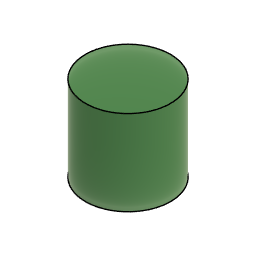
TrueTip Assembly (Autodesk Fusion 360 archive; units mm, degrees)
design "Traceline Dummy"
Autodesk Fusion 360 part; units mm, degrees
(part 1 of 3)
sketch "Sketch1" plane through (0, 0, 0) normal (0, 0, 1) x (1, 0, 0)
  circle A0 centre (0, 0) radius 0.05
  dimension "d1" = 0.1
  constraint coincident A0.centre origin
  measures "d1" diameter of A0
extrude "Extrude1" add sketch "Sketch1" along normal blind 0.1

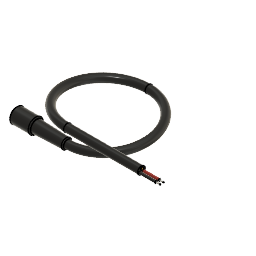
design "PE2 - 3-Pin Male Waterproof Connector (cut, coiled)"
Autodesk Fusion 360 part; units mm, degrees
sketch "Sketch1" plane through (0, 0, 0) normal (1, 0, 0) x (0, 1, 0)
  circle A0 centre (0, 0) radius 3.683
  circle A1 centre (0, 0) radius 3.175
  dimension "d1" = 7.366
  dimension "d2" = 6.35
  constraint coincident A0.centre A1.centre
  constraint concentric A0 A1
  measures "d1" diameter of A0
  measures "d2" diameter of A1
extrude "Extrude1" add sketch "Sketch1" along normal blind 10 contours A0 | A1 makes body 1
extrude "Extrude2" cut sketch "Sketch1" along normal blind 8 contours A1 bodies 1
sketch "Sketch2" plane through (0, 0, 0) normal (0, 1, 0) x (1, 0, 0)
  line L0 (10, 0) -> (10, -3)
  line L1 (10, -3) -> (25, -2.5)
  line L2 (25, -2.5) -> (25, 0)
  line L3 (25, 0) -> (10, 0)
  dimension "d7" = 3
  dimension "d46" = 15
  dimension "d47" = 88.091
  dimension "d48" = 10
  constraint vertical L0
  constraint vertical L2
  constraint perpendicular L0 L3
  constraint horizontal origin L0.start
  measures "d7" distance of L0.start L0.end
  measures "d46" distance of L0 L2
  measures "d47" angle of L0 L1
  measures "d48" distance of origin L0
revolve "Revolve1" add sketch "Sketch2" angle 360 about axis through (1.75, 0, 0) along (1, 0, 0) bodies 1
fillet "Fillet1" radius 0.5 3 edges at (0, -3.4338, -1.3318) (10, -3.4338, -1.3318) (25, -0.904, -2.3308) on bodies 1
sketch "Sketch4" plane through (8, 0, 0) normal (1, 0, 0) x (0, 1, 0)
  line L0 (0, 1.5) -> (-1.299, -0.75) construction
  line L1 (-1.299, -0.75) -> (1.299, -0.75) construction
  line L2 (1.299, -0.75) -> (0, 1.5) construction
  circle A0 centre (0, 1.5) radius 0.5
  circle A1 centre (-1.299, -0.75) radius 0.5
  circle A2 centre (1.299, -0.75) radius 0.5
  dimension "d15" = 1.5
  dimension "d16" = 1
  dimension "d17" = 1
  dimension "d18" = 1
  constraint coincident L0.start L2.end
  constraint coincident L0.end L1.start
  constraint coincident L1.end L2.start
  constraint horizontal L1
  measures "d15" distance of L0.start origin
  measures "d16" diameter of A0
  measures "d17" diameter of A1
  measures "d18" diameter of A2
extrude "Extrude4" add sketch "Sketch4" against normal blind 8 separate body makes body 2 at (2.6667, 0.4975, 1.4502) makes body 3 at (2.6667, 1.7966, -0.7998) makes body 4 at (2.6667, -0.8015, -0.7998)
fillet "Fillet2" radius 0.1 3 edges at (0, -0.4662, 1.6808) (0, 0.8329, -0.5692) (0, -1.7652, -0.5692) on bodies 2 3 4
sketch "Sketch3" plane through (25, 0, 0) normal (1, 0, 0) x (0, 1, 0)
  circle A0 centre (0, 0) radius 1.905
  circle A1 centre (0, 0) radius 2.0164
  dimension "d9" = 3.81
  constraint coincident A0.centre A1.centre
  measures "d9" diameter of A0
sketch "Sketch5" plane through (0, 0, 0) normal (0, 0, 1) x (1, 0, 0)
  arc A0 through (25, 0, 0) (45, 19.9239, 1.7431) (25, 39.8478, 3.4862)
  arc A1 through (25, 39.8478, 3.4862) (5, 19.9239, 5.2293) (25, 0, 6.9725)
  dimension "d42" = 40
  dimension "d49" = 3.4862
  dimension "d50" = 6.9725
sweep "Sweep1" add profiles "Sketch3" path "Sketch5" along A0 A1 section 1 contours A0 bodies 1
extrude "Extrude5" add 1 faces at (25, -0.5824, 7.9009) along direction (1, 0, 0) blind 36.2 on bodies 1 bodies 1
sketch "Sketch6" plane through (61.2, 0, 0) normal (1, 0, 0) x (0, 1, 0)
  line L0 (0, 7.9725) -> (-0.866, 6.4725) construction
  line L1 (-0.866, 6.4725) -> (0.866, 6.4725) construction
  line L2 (0.866, 6.4725) -> (0, 7.9725) construction
  circle A0 centre (0, 7.9725) radius 0.625
  circle A1 centre (0.866, 6.4725) radius 0.625
  circle A2 centre (-0.866, 6.4725) radius 0.625
  circle A3 centre (0, 6.9725) radius 1.905
  point P0 (0, 6.9725)
  dimension "d31" = 1
  dimension "d32" = 1.25
  dimension "d33" = 1.25
  dimension "d34" = 1.25
  constraint coincident L0.start L2.end
  constraint coincident L1.end L2.start
  constraint coincident L0.end L1.start
  constraint coincident P0 A3.centre
  constraint vertical L0.start P0
  measures "d31" distance of L0.start P0
  measures "d32" diameter of A0
  measures "d33" diameter of A1
  measures "d34" diameter of A2
extrude "Extrude6" add sketch "Sketch6" along normal blind 8 separate body contours A1 | A2 makes body 5 at (63.8667, -0.2441, 6.4102) makes body 6 at (63.8667, 1.4879, 6.4102)
sketch "Sketch7" plane through (69.2, 0, 0) normal (1, 0, 0) x (0, 1, 0)
  circle A0 centre (0, 7.9725) radius 0.375
  circle A1 centre (-0.866, 6.4725) radius 0.625
  circle A2 centre (0.866, 6.4725) radius 0.625
  dimension "d43" = 0.75
  dimension "d51" = 1.5
  dimension "d52" = 0.866
  measures "d43" diameter of A0
  measures "d51" vertical distance of A0.centre A1.centre
  measures "d52" horizontal distance of A0.centre A1.centre
sketch "Sketch8" plane through (69.2, 0, 0) normal (1, 0, 0) x (0, 1, 0)
  circle A0 centre (0.866, 6.4725) radius 0.625
  circle A1 centre (0.866, 6.4725) radius 0.375
  dimension "d37" = 0.75
  constraint concentric A0 A1
  measures "d37" diameter of A1
sketch "Sketch9" plane through (69.2, 0, 0) normal (1, 0, 0) x (0, 1, 0)
  circle A0 centre (-0.866, 6.4725) radius 0.625
  circle A1 centre (-0.866, 6.4725) radius 0.375
  dimension "d38" = 0.75
  constraint concentric A0 A1
  measures "d38" diameter of A1
extrude "Extrude7" add sketch "Sketch8" sketch "Sketch9" along normal blind 2 separate body contours A1 of sketch 2 contours A1 makes body 7 at (69.8667, 1.2392, 6.4351) makes body 8 at (69.8667, -0.4929, 6.4351)
extrude "Extrude8" add sketch "Sketch6" along normal blind 0.5 separate body contours A0 makes body 9

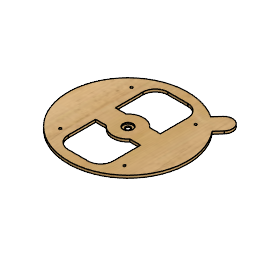
design "LB3 - Bucket Adapter"
Autodesk Fusion 360 part; units mm, degrees
sketch "Sketch1" plane through (0, 0, 0) normal (0, 0, 1) x (1, 0, 0)
  circle A0 centre (-64.5, 71.5) radius 2.25
  circle A1 centre (64.5, 71.5) radius 2.25
  circle A2 centre (-64.5, -71.5) radius 2.25
  circle A3 centre (64.5, -71.5) radius 2.25
  line L0 (20, 100) -> (-20, 100)
  line L1 (-20, -100) -> (20, -100)
  arc A4 (-20, 100) -> (-45, 75) centre (-20, 75) ccw
  arc A5 (45, 75) -> (20, 100) centre (20, 75) ccw
  arc A6 (20, -100) -> (45, -75) centre (20, -75) ccw
  arc A7 (-45, -75) -> (-20, -100) centre (-20, -75) ccw
  line L2 (45, 20) -> (-45, -20) construction
  circle A8 centre (0, 0) radius 5
  line L3 (64.5, 71.5) -> (-64.5, 71.5) construction
  line L4 (-64.5, 71.5) -> (-64.5, -71.5) construction
  line L5 (-64.5, -71.5) -> (64.5, -71.5) construction
  line L6 (64.5, -71.5) -> (64.5, 71.5) construction
  line L7 (64.5, 71.5) -> (-64.5, -71.5) construction
  line L8 (-64.5, 71.5) -> (64.5, -71.5) construction
  line L9 (45, 20) -> (23.6854, 20)
  line L10 (-23.6854, 20) -> (-45, 20)
  line L11 (-45, 75) -> (-45, 20)
  line L12 (-45, -20) -> (-45, -75)
  arc A9 (-23.6854, -20) -> (23.6854, -20) centre (0, 0) ccw
  arc A10 (23.6854, 20) -> (-23.6854, 20) centre (0, 0) ccw
  line L13 (45, -75) -> (45, -20)
  line L14 (45, 20) -> (45, 75)
  line L15 (-45, 20) -> (4.5691, -2.0307) construction
  line L16 (28.3282, -12.5903) -> (45, -20) construction
  line L17 (-45, -20) -> (-23.6854, -20)
  line L18 (23.6854, -20) -> (45, -20)
  line L19 (91.0962, 100.9826) -> (104.4615, 88.9257) construction
  line L20 (91.0962, 100.9826) -> (77.7308, 113.0394) construction
  line L21 (104.4615, 88.9257) -> (92.8349, 76.0373)
  line L22 (77.7308, 113.0394) -> (66.1042, 100.151)
  arc A11 (104.4615, 88.9257) -> (77.7308, 113.0394) centre (91.0962, 100.9826) ccw
  arc A12 (66.1042, 100.151) -> (92.8349, 76.0373) centre (0, 0) ccw
  dimension "d14" = 4.5
  dimension "d15" = 4.5
  dimension "d16" = 4.5
  dimension "d17" = 4.5
  dimension "d20" = 240
  dimension "d21" = 25
  dimension "d23" = 40
  dimension "d24" = 10
  dimension "d25" = 62
  dimension "d26" = 129
  dimension "d27" = 143
  dimension "d29" = 36
  dimension "d33" = 45
  dimension "d34" = 100
  dimension "d35" = 100
  dimension "d36" = 149.4615
  dimension "d37" = 132.054
  dimension "d38" = 213.0394
  dimension "d39" = 18.2443
  dimension "d40" = 18
  constraint horizontal L0
  constraint perpendicular L0 L11
  constraint parallel L0 L1
  constraint parallel L11 L13
  constraint tangent L0 A4
  constraint tangent A4 L11
  constraint tangent A5 L13
  constraint tangent L0 A5
  constraint equal A4 A5
  constraint tangent L1 A6
  constraint tangent A6 L13
  constraint equal A4 A6
  constraint tangent A7 L11
  constraint tangent L1 A7
  constraint equal A4 A7
  constraint horizontal L9
  constraint parallel L9 L17
  constraint coincident L2 A8.centre
  constraint coincident A8.centre L15
  constraint coincident A8.centre A9.centre
  constraint concentric A8 A12
  constraint horizontal L3
  constraint perpendicular L3 L4
  constraint parallel L3 L5
  constraint parallel L4 L6
  constraint coincident L7 A8.centre
  constraint coincident L8 A8.centre
  constraint collinear L9 L10
  constraint coincident L10.start A9
  constraint coincident L9.end A9
  constraint collinear L11 L12
  constraint coincident L16.start L15
  constraint concentric A9 A10
  constraint collinear L13 L14
  constraint coincident A8 L15.end
  constraint collinear L15 L16
  constraint coincident A9.end L17
  constraint collinear L17 L18
  constraint coincident L19.start L20.start
  constraint tangent L21 A11
  constraint tangent L22 A11
  constraint concentric A8 A9
  constraint coincident A2.centre L4.end
  constraint coincident A1.centre L3.start
  constraint coincident A3.centre L5.end
  constraint coincident A0.centre L3.end
  measures "d14" diameter of A0
  measures "d15" diameter of A1
  measures "d16" diameter of A2
  measures "d17" diameter of A3
  measures "d20" diameter of A12
  measures "d21" radius of A4
  measures "d23" distance of L10.end L2.end
  measures "d24" diameter of A8
  measures "d25" diameter of A9
  measures "d26" distance of A2.centre A3.centre
  measures "d27" distance of A0.centre A2.centre
  measures "d29" diameter of A11
  measures "d33" distance of A8.centre L11
  measures "d34" distance of A8.centre L1
  measures "d35" distance of A8.centre L0
  measures "d36" distance of L11 L19.end
  measures "d37" angle of L3 L21
  measures "d38" distance of L1 L20.end
  measures "d39" distance of L13.end L16.start
  measures "d40" distance of L7 L21
extrude "Extrude1" add sketch "Sketch1" along normal blind 5.2
sketch "Sketch4" plane through (0, 0, 5.2) normal (0, 0, 1) x (-1, 0, 0)
  circle A0 centre (-64.5, 71.5) radius 2.25
  circle A1 centre (64.5, 71.5) radius 2.25
  line L0 (-45, -20) -> (-23.6854, -20)
  arc A2 (-23.6854, -20) -> (23.6854, -20) centre (0, 0) ccw
  line L1 (23.6854, -20) -> (45, -20)
  line L2 (45, -20) -> (45, -75)
  arc A3 (20, -100) -> (45, -75) centre (20, -75) ccw
  line L3 (20, -100) -> (-20, -100)
  arc A4 (-45, -75) -> (-20, -100) centre (-20, -75) ccw
  line L4 (-45, -75) -> (-45, -20)
  circle A5 centre (64.5, -71.5) radius 2.25
  circle A6 centre (0, 0) radius 5
  line L5 (45, 75) -> (45, 20)
  line L6 (45, 20) -> (23.6854, 20)
  arc A7 (23.6854, 20) -> (-23.6854, 20) centre (0, 0) ccw
  line L7 (-23.6854, 20) -> (-45, 20)
  line L8 (-45, 20) -> (-45, 75)
  arc A8 (-20, 100) -> (-45, 75) centre (-20, 75) ccw
  line L9 (-20, 100) -> (20, 100)
  arc A9 (45, 75) -> (20, 100) centre (20, 75) ccw
  circle A10 centre (-64.5, -71.5) radius 2.25
  arc A11 (-104.4615, -88.9257) -> (-77.7308, -113.0394) centre (-91.0962, -100.9826) ccw
  line L10 (-77.7308, -113.0394) -> (-66.1042, -100.151)
  arc A12 (-66.1042, -100.151) -> (-92.8349, -76.0373) centre (0, 0) ccw
  line L11 (-92.8349, -76.0373) -> (-104.4615, -88.9257)
  circle A13 centre (0, 0) radius 10
  dimension "d30" = 20
  constraint concentric A2 A13
  measures "d30" diameter of A13
extrude "Extrude3" cut sketch "Sketch4" against normal blind 2.6 contours A13
equation "d31 = ( -5.2 / 2 ) * 1 mm"

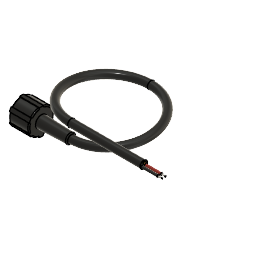
design "FA8 - 3-Pin Female Waterproof Connector (coiled)"
Autodesk Fusion 360 part; units mm, degrees
sketch "Sketch1" plane through (0, 0, 0) normal (1, 0, 0) x (0, 1, 0)
  circle A0 centre (0, 0) radius 6.35
  circle A1 centre (0, 0) radius 5.08
  dimension "d1" = 12.7
  dimension "d2" = 10.16
  constraint coincident A0.centre A1.centre
  constraint concentric A0 A1
  measures "d1" diameter of A0
  measures "d2" diameter of A1
extrude "Extrude1" add sketch "Sketch1" along normal blind 10 contours A0 | A1 makes body 1
extrude "Extrude2" cut sketch "Sketch1" along normal blind 8 contours A1 bodies 1
sketch "Sketch2" plane through (0, 0, 0) normal (0, 1, 0) x (1, 0, 0)
  line L0 (10, 0) -> (10, -3)
  line L1 (10, -3) -> (25, -2.5)
  line L2 (25, -2.5) -> (25, 0)
  line L3 (25, 0) -> (10, 0)
  dimension "d7" = 3
  constraint vertical L0
  constraint vertical L2
  constraint perpendicular L0 L3
  measures "d7" distance of L0.start L0.end
revolve "Revolve1" add sketch "Sketch2" angle 360 about axis through (1.75, 0, 0) along (1, 0, 0) bodies 1
fillet "Fillet1" radius 0.5 3 edges at (0, -5.9203, -2.2963) (10, -5.9203, -2.2963) (25, -0.904, -2.3308) on bodies 1
sketch "Sketch4" plane through (8, 0, 0) normal (1, 0, 0) x (0, 1, 0)
  line L0 (0, 1.5) -> (-1.299, -0.75) construction
  line L1 (-1.299, -0.75) -> (1.299, -0.75) construction
  line L2 (1.299, -0.75) -> (0, 1.5) construction
  circle A0 centre (0, 1.5) radius 0.5
  circle A1 centre (-1.299, -0.75) radius 0.5
  circle A2 centre (1.299, -0.75) radius 0.5
  circle A3 centre (0, 0) radius 2.25
  dimension "d15" = 1.5
  dimension "d16" = 1
  dimension "d17" = 1
  dimension "d18" = 1
  dimension "d43" = 4.5
  constraint coincident A3.centre origin
  constraint coincident L0.start L2.end
  constraint coincident L0.end L1.start
  constraint coincident L1.end L2.start
  measures "d15" distance of L0.start A3.centre
  measures "d16" diameter of A0
  measures "d17" diameter of A1
  measures "d18" diameter of A2
  measures "d43" diameter of A3
extrude "Extrude8" add sketch "Sketch4" against normal blind 8 bodies 1
sketch "Sketch10" plane through (0, 0, 0) normal (0, 0, 1) x (1, 0, 0)
  line L0 (10, -1) -> (0, -1)
  line L1 (0, 1) -> (10, 1)
  line L2 (10, 1) -> (10, -1)
  line L3 (10, -1) -> (0, 0) construction
  line L4 (0, 0) -> (10, 1) construction
  line L5 (0, -1) -> (0, 1)
  constraint horizontal L0
  constraint parallel L0 L1
  constraint coincident L3 L4.start
  constraint coincident L4 L3.end
  constraint coincident L3.end L4.start
extrude "Extrude9" add sketch "Sketch10" along normal blind 1 from surface at 5.5 bodies 1
pattern_circular "C-Pattern1" count 6 over 360 about axis through (1.75, 0, 0) along (1, 0, 0) of "Extrude9"
sketch "Sketch3" plane through (25, 0, 0) normal (1, 0, 0) x (0, 1, 0)
  circle A0 centre (0, 0) radius 1.905
  circle A1 centre (0, 0) radius 2.0164
  dimension "d9" = 3.81
  constraint coincident A0.centre A1.centre
  measures "d9" diameter of A0
sketch "Sketch5" plane through (0, 0, 0) normal (0, 0, 1) x (1, 0, 0)
  arc A0 through (25, 0, 0) (45, 19.9239, 1.7431) (25, 39.8478, 3.4862)
  arc A1 through (25, 39.8478, 3.4862) (5, 19.9239, 5.2293) (25, 0, 6.9725)
  dimension "d42" = 40
sweep "Sweep1" add profiles "Sketch3" path "Sketch5" along A0 A1 section 1 contours A0 bodies 1
extrude "Extrude5" add 1 faces at (25, -0.7992, 7.2336) along direction (1, 0, 0) blind 36.2 on bodies 1 bodies 1
sketch "Sketch6" plane through (61.2, 0, 0) normal (1, 0, 0) x (0, 1, 0)
  line L0 (0, 7.9725) -> (-0.866, 6.4725) construction
  line L1 (-0.866, 6.4725) -> (0.866, 6.4725) construction
  line L2 (0.866, 6.4725) -> (0, 7.9725) construction
  circle A0 centre (0, 7.9725) radius 0.625
  circle A1 centre (0.866, 6.4725) radius 0.625
  circle A2 centre (-0.866, 6.4725) radius 0.625
  circle A3 centre (0, 6.9725) radius 1.905
  point P0 (0, 6.9725)
  dimension "d31" = 1
  dimension "d32" = 1.25
  dimension "d33" = 1.25
  dimension "d34" = 1.25
  constraint coincident L0.start L2.end
  constraint coincident L1.end L2.start
  constraint coincident L0.end L1.start
  measures "d31" distance of L0.start P0
  measures "d32" diameter of A0
  measures "d33" diameter of A1
  measures "d34" diameter of A2
extrude "Extrude6" add sketch "Sketch6" along normal blind 8 separate body contours A1 | A2 makes body 2 at (63.8667, -0.2441, 6.4102) makes body 3 at (63.8667, 1.4879, 6.4102)
sketch "Sketch7" plane through (69.2, 0, 0) normal (1, 0, 0) x (0, 1, 0)
  circle A0 centre (0, 7.9725) radius 0.375
  circle A1 centre (0.866, 6.4725) radius 0.625
  circle A2 centre (-0.866, 6.4725) radius 0.625
  dimension "d52" = 0.75
  measures "d52" diameter of A0
sketch "Sketch8" plane through (69.2, 0, 0) normal (1, 0, 0) x (0, 1, 0)
  circle A0 centre (0.866, 6.4725) radius 0.625
  circle A1 centre (0.866, 6.4725) radius 0.375
  dimension "d37" = 0.75
  constraint concentric A0 A1
  measures "d37" diameter of A1
sketch "Sketch9" plane through (69.2, 0, 0) normal (1, 0, 0) x (0, 1, 0)
  circle A0 centre (-0.866, 6.4725) radius 0.625
  circle A1 centre (-0.866, 6.4725) radius 0.375
  dimension "d38" = 0.75
  constraint concentric A0 A1
  measures "d38" diameter of A1
extrude "Extrude7" add sketch "Sketch8" sketch "Sketch9" along normal blind 2 separate body contours A1 of sketch 2 contours A1 makes body 4 at (69.8667, 1.2392, 6.4351) makes body 5 at (69.8667, -0.4929, 6.4351)
extrude "Extrude10" add sketch "Sketch6" along normal blind 0.5 separate body contours A0 makes body 6

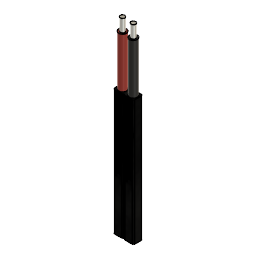
design "Wire End (FA1)"
Autodesk Fusion 360 part; units mm, degrees
sketch "Sketch1" plane through (0, 0, 0) normal (0, 0, 1) x (1, 0, 0)
  line L0 (1.625, -0.55) -> (1.625, 0.55)
  arc A0 (-1.625, -0.55) -> (-1.425, -0.75) centre (-1.425, -0.55) ccw
  line L1 (-1.625, 0.55) -> (-1.625, -0.55)
  arc A1 (-1.425, 0.75) -> (-1.625, 0.55) centre (-1.425, 0.55) ccw
  arc A2 (1.425, -0.75) -> (1.625, -0.55) centre (1.425, -0.55) ccw
  line L2 (1.625, -0.75) -> (-1.625, 0.75) construction
  line L3 (-1.625, -0.75) -> (1.625, 0.75) construction
  arc A3 (1.625, 0.55) -> (1.425, 0.75) centre (1.425, 0.55) ccw
  arc A4 (-0.1231, 0.6643) -> (0.1231, 0.6643) centre (0, 0.75) ccw
  line L4 (1.425, 0.75) -> (0.2872, 0.75)
  line L5 (-0.2872, 0.75) -> (-1.425, 0.75)
  arc A5 (0.1129, -0.6643) -> (-0.1333, -0.6643) centre (-0.0102, -0.75) ccw
  line L6 (-1.425, -0.75) -> (-0.2975, -0.75)
  line L7 (0.277, -0.75) -> (1.425, -0.75)
  arc A6 (-0.1231, 0.6643) -> (-0.2872, 0.75) centre (-0.2872, 0.55) ccw
  arc A7 (0.2872, 0.75) -> (0.1231, 0.6643) centre (0.2872, 0.55) ccw
  arc A8 (0.1129, -0.6643) -> (0.277, -0.75) centre (0.277, -0.55) ccw
  arc A9 (-0.2975, -0.75) -> (-0.1333, -0.6643) centre (-0.2975, -0.55) ccw
  dimension "d15" = 3.25
  dimension "d16" = 1.5
  dimension "d17" = 0.2
  dimension "d18" = 0.2
  dimension "d19" = 0.3
  dimension "d20" = 0.3
  dimension "d21" = 0.2
  constraint perpendicular L0 L6
  constraint parallel L4 L6
  constraint parallel L0 L1
  constraint coincident origin L3
  constraint coincident origin L2
  constraint coincident L2.start L6
  constraint coincident L2.start L0
  constraint tangent A2 L6
  constraint tangent L0 A2
  constraint coincident L3.start L1
  constraint coincident L3.start L6
  constraint tangent A0 L1
  constraint tangent A0 L6
  constraint equal A0 A2
  constraint coincident L2.end L1
  constraint coincident L2.end L4
  constraint tangent L1 A1
  constraint tangent A1 L4
  constraint equal A1 A2
  constraint coincident L3.end L4
  constraint coincident L3.end L0
  constraint tangent A3 L4
  constraint tangent L0 A3
  constraint collinear L4 L5
  constraint coincident A4.centre L4
  constraint collinear L6 L7
  constraint coincident A5.centre L6
  constraint tangent A4 A6
  constraint tangent L5 A6
  constraint tangent A4 A7
  constraint tangent L4 A7
  constraint equal A6 A7
  constraint tangent A5 A8
  constraint tangent L7 A8
  constraint equal A6 A8
  constraint tangent A5 A9
  constraint tangent L6 A9
  constraint equal A6 A9
  measures "d15" distance of L3.end L2.end
  measures "d16" distance of L3.end L2.start
  measures "d17" radius of A2
  measures "d18" radius of A3
  measures "d19" diameter of A4
  measures "d20" diameter of A5
  measures "d21" radius of A6
extrude "Extrude1" add sketch "Sketch1" along normal blind 20 makes body 1
sketch "Sketch2" plane through (0, 0, 20) normal (0, 0, 1) x (-1, 0, 0)
  line L0 (0, 0) -> (-0.866, 0) construction
  line L1 (0, 0) -> (0.866, 0) construction
  circle A0 centre (-0.866, 0) radius 0.625
  circle A1 centre (0.866, 0) radius 0.625
  line L2 (0.2872, -0.75) -> (1.425, -0.75)
  arc A2 (1.425, -0.75) -> (1.625, -0.55) centre (1.425, -0.55) ccw
  line L3 (1.625, -0.55) -> (1.625, 0.55)
  arc A3 (1.625, 0.55) -> (1.425, 0.75) centre (1.425, 0.55) ccw
  line L4 (1.425, 0.75) -> (0.2975, 0.75)
  arc A4 (-1.425, 0.75) -> (-1.625, 0.55) centre (-1.425, 0.55) ccw
  line L5 (-1.625, 0.55) -> (-1.625, -0.55)
  arc A5 (-1.625, -0.55) -> (-1.425, -0.75) centre (-1.425, -0.55) ccw
  arc A6 (0.1231, -0.6643) -> (0.2872, -0.75) centre (0.2872, -0.55) ccw
  arc A7 (0.2975, 0.75) -> (0.1333, 0.6643) centre (0.2975, 0.55) ccw
  arc A8 (-0.1129, 0.6643) -> (0.1333, 0.6643) centre (0.0102, 0.75) ccw
  arc A9 (-0.1129, 0.6643) -> (-0.277, 0.75) centre (-0.277, 0.55) ccw
  line L6 (-0.277, 0.75) -> (-1.425, 0.75)
  line L7 (-1.425, -0.75) -> (-0.2872, -0.75)
  arc A10 (-0.2872, -0.75) -> (-0.1231, -0.6643) centre (-0.2872, -0.55) ccw
  arc A11 (0.1231, -0.6643) -> (-0.1231, -0.6643) centre (0, -0.75) ccw
  dimension "d5" = 0.866
  dimension "d6" = 0.866
  dimension "d7" = 1.25
  dimension "d8" = 1.25
  constraint coincident L0.start L1.start
  constraint horizontal L0
  constraint parallel L0 L1
  constraint coincident L0.end A0.centre
  constraint coincident L1.end A1.centre
  measures "d5" distance of L0.start L0.end
  measures "d6" distance of L0.start L1.end
  measures "d7" diameter of A0
  measures "d8" diameter of A1
extrude "Extrude2" add sketch "Sketch2" along normal blind 8 separate body contours A0 | A1 makes body 2 at (-1.4879, 0.0622, 22.6667) makes body 3 at (0.2441, 0.0622, 22.6667)
sketch "Sketch3" plane through (0, 0, 28) normal (0, 0, 1) x (-1, 0, 0)
  circle A0 centre (0.866, 0) radius 0.625
  circle A1 centre (0.866, 0) radius 0.375
  dimension "d11" = 0.75
  constraint concentric A0 A1
  measures "d11" diameter of A1
sketch "Sketch4" plane through (0, 0, 28) normal (0, 0, 1) x (-1, 0, 0)
  circle A0 centre (-0.866, 0) radius 0.625
  circle A1 centre (-0.866, 0) radius 0.375
  dimension "d12" = 0.75
  constraint concentric A0 A1
  measures "d12" diameter of A1
extrude "Extrude3" add sketch "Sketch4" sketch "Sketch3" along normal blind 2 separate body contours A1 of sketch 2 contours A1 makes body 4 at (0.4929, 0.0373, 28.6667) makes body 5 at (-1.2392, 0.0373, 28.6667)
equation "d5 = 1.73205081 mm / 2"
equation "d6 = 1.73205081 mm / 2"

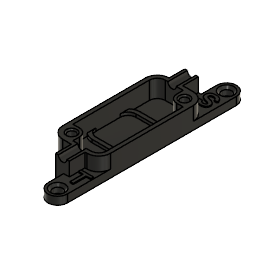
design "PE3 - PCB Case"
Autodesk Fusion 360 part; units mm, degrees
sketch "Sketch1" plane through (0, 0, 0) normal (0, 0, 1) x (1, 0, 0)
  line L0 (6.2013, 10.25) -> (-6.2012, 10.25)
  line L1 (-10.25, 6.2013) -> (-10.25, -6.2012)
  line L2 (-6.2012, -10.25) -> (6.2013, -10.25)
  line L3 (10.25, -6.2012) -> (10.25, 6.2012)
  line L4 (10.25, 10.25) -> (-10.25, -10.25) construction
  line L5 (-10.25, 10.25) -> (10.25, -10.25) construction
  arc A0 (-6.2012, 10.25) -> (-10.25, 6.2013) centre (-6.2013, 6.2013) ccw
  arc A1 (10.25, 6.2012) -> (6.2013, 10.25) centre (6.2012, 6.2012) ccw
  arc A2 (-10.25, -6.2012) -> (-6.2012, -10.25) centre (-6.2013, -6.2013) ccw
  arc A3 (6.2013, -10.25) -> (10.25, -6.2012) centre (6.2013, -6.2013) ccw
  line L6 (-12.25, 6.2013) -> (-12.25, -6.2013)
  arc A4 (-12.25, -6.2012) -> (-6.2012, -12.25) centre (-6.2013, -6.2013) ccw
  line L7 (-6.2012, -12.25) -> (6.2013, -12.25)
  arc A5 (6.2013, -12.25) -> (12.25, -6.2012) centre (6.2013, -6.2013) ccw
  line L8 (12.25, -6.2012) -> (12.25, 6.2012)
  arc A6 (12.25, 6.2012) -> (6.2013, 12.25) centre (6.2012, 6.2012) ccw
  line L9 (6.2013, 12.25) -> (-6.2012, 12.25)
  arc A7 (-6.2012, 12.25) -> (-12.25, 6.2013) centre (-6.2013, 6.2013) ccw
  dimension "d1" = 20.5
  dimension "d2" = 20.5
  dimension "d3" = 4.0488
  dimension "d4" = 4.0488
  dimension "d5" = 4.0488
  dimension "d6" = 4.0488
  dimension "d7" = 2
  constraint horizontal L0
  constraint perpendicular L0 L1
  constraint parallel L0 L2
  constraint parallel L1 L3
  constraint coincident L4 origin
  constraint coincident L5 origin
  constraint coincident L5.start L0
  constraint coincident L5.start L1
  constraint tangent L0 A0
  constraint tangent L1 A0
  constraint coincident L4.start L0
  constraint coincident L4.start L3
  constraint tangent L0 A1
  constraint tangent L3 A1
  constraint coincident L4.end L2
  constraint coincident L4.end L1
  constraint tangent L2 A2
  constraint tangent L1 A2
  constraint coincident L5.end L3
  constraint coincident L5.end L2
  constraint tangent L3 A3
  constraint tangent L2 A3
  measures "d1" distance of L4.start L5.start
  measures "d2" distance of L4.start L5.end
  measures "d3" radius of A0
  measures "d4" radius of A1
  measures "d5" radius of A2
  measures "d6" radius of A3
extrude "Extrude1" add sketch "Sketch1" along normal blind 6 contours L0 L1 L2 L3 A0 A1 A2 A3 | L6 A4 L7 A5 L8 A6 L9 A7
extrude "Extrude2" add sketch "Sketch1" along normal blind 1.5 from surface at 6
sketch "Sketch10" plane through (0, 0, 0) normal (0, 0, 1) x (1, 0, 0)
  line L0 (7.2501, -43.2789) -> (7.2501, 43.2211) construction
  line L1 (7.2501, -0.0289) -> (8.1135, -0.0289) construction
  circle A0 centre (7.2501, 43.2211) radius 2.5
  circle A1 centre (7.2501, -43.2789) radius 2.5
  arc A2 (2.2502, -43.2493) -> (12.25, -43.25) centre (7.2501, -43.2789) ccw
  arc A3 (12.25, 43.1922) -> (2.2502, 43.1914) centre (7.2501, 43.2211) ccw
  line L2 (2.2502, 43.1914) -> (2.2502, -43.3086)
  line L3 (12.25, -43.25) -> (12.25, 43.25)
  dimension "d42" = 86.5
  dimension "d43" = 5
  dimension "d44" = 5
  dimension "d45" = 10
  dimension "d46" = 10
  dimension "d134" = 0.0289
  dimension "d135" = 7.2501
  dimension "d136" = 0.8634
  constraint midpoint L0 L1.start
  constraint perpendicular L0 L1
  constraint coincident L0.end A0.centre
  constraint coincident L0.start A1.centre
  constraint concentric A1 A2
  constraint concentric A0 A3
  constraint parallel L0 L2
  constraint coincident A2 L2.end
  constraint coincident L2 A2.start
  constraint vertical L3
  constraint coincident L3 A3.start
  constraint coincident A3 L3.end
  constraint parallel L0 L3
  constraint equal L0 L2
  constraint equal L0 L3
  measures "d42" distance of L0.start L0.end
  measures "d43" diameter of A0
  measures "d44" diameter of A1
  measures "d45" diameter of A2
  measures "d46" diameter of A3
  measures "d134" distance of origin L1
  measures "d135" distance of origin L0
  measures "d136" distance of L0 L1.end
extrude "Extrude10" add sketch "Sketch10" along normal blind 4
chamfer "Chamfer1" distance 1.25 angle 45 2 edges at (6.346, -45.6097, 4) (6.346, 40.8903, 4)
sketch "Sketch12" plane through (0, 0, 0) normal (0, 0, -1) x (1, 0, 0)
  circle A0 centre (7.2501, 43.2789) radius 2.5
  circle A1 centre (7.2501, -43.2211) radius 2.5
  line L0 (2.2502, 12.25) -> (-6.2012, 12.25)
  arc A2 (-6.2013, 12.25) -> (-12.25, 6.2012) centre (-6.2013, 6.2013) ccw
  line L1 (-12.25, 6.2012) -> (-12.25, -6.2013)
  arc A3 (-12.25, -6.2013) -> (-6.2012, -12.25) centre (-6.2013, -6.2013) ccw
  line L2 (2.2502, -12.25) -> (2.2502, -43.1914)
  arc A4 (2.2502, -43.1914) -> (12.25, -43.25) centre (7.2501, -43.2211) ccw
  line L3 (12.25, -43.25) -> (12.25, 43.25)
  arc A5 (12.25, 43.25) -> (2.2502, 43.3086) centre (7.2501, 43.2789) ccw
  line L4 (10.25, -21.2012) -> (10.25, 21.2013)
  arc A6 (-6.2013, 25.25) -> (-10.25, 21.2013) centre (-6.2013, 21.2013) ccw
  arc A7 (-12.25, -21.2012) -> (-6.2013, -27.25) centre (-6.2013, -21.2012) ccw
  arc A8 (6.2013, -25.25) -> (10.25, -21.2012) centre (6.2013, -21.2012) ccw
  line L5 (-10.25, 25.25) -> (10.25, -25.25) construction
  line L6 (10.25, 25.25) -> (-10.25, -25.25) construction
  line L7 (-12.25, 21.2012) -> (-12.25, -21.2012)
  line L8 (-10.25, 21.2013) -> (-10.25, -21.2012)
  arc A9 (12.25, 21.2013) -> (6.2013, 27.25) centre (6.2012, 21.2013) ccw
  arc A10 (-6.2012, 27.25) -> (-12.25, 21.2012) centre (-6.2013, 21.2013) ccw
  line L9 (-6.2013, -25.25) -> (6.2013, -25.25)
  line L10 (6.2012, 25.25) -> (-6.2013, 25.25)
  line L11 (12.25, -21.2012) -> (12.25, 21.2013)
  arc A11 (10.25, 21.2013) -> (6.2012, 25.25) centre (6.2012, 21.2013) ccw
  arc A12 (-10.25, -21.2012) -> (-6.2013, -25.25) centre (-6.2013, -21.2012) ccw
  arc A13 (6.2012, -27.25) -> (12.25, -21.2012) centre (6.2013, -21.2012) ccw
  line L12 (-6.2013, -27.25) -> (6.2012, -27.25)
  line L13 (6.2013, 27.25) -> (-6.2012, 27.25)
  line L14 (-6.2012, -12.25) -> (2.2502, -12.25)
  line L15 (2.2502, 43.3086) -> (2.2502, 12.25)
  dimension "d77" = 2
  dimension "d78" = 20.5
  dimension "d79" = 50.5
  dimension "d80" = 4.0488
  dimension "d81" = 4.0488
  dimension "d82" = 4.0488
  dimension "d83" = 4.0488
  constraint horizontal L10
  constraint perpendicular L8 L10
  constraint parallel L9 L10
  constraint parallel L4 L8
  constraint coincident origin L6
  constraint coincident origin L5
  constraint coincident L5.start L10
  constraint coincident L5.start L8
  constraint tangent A6 L10
  constraint tangent A6 L8
  constraint coincident L6.start L10
  constraint coincident L6.start L4
  constraint tangent L10 A11
  constraint tangent L4 A11
  constraint coincident L6.end L9
  constraint coincident L6.end L8
  constraint tangent L9 A12
  constraint tangent L8 A12
  constraint coincident L5.end L4
  constraint coincident L5.end L9
  constraint tangent L4 A8
  constraint tangent A8 L9
  measures "d78" distance of L5.start L6.start
  measures "d79" distance of L5.end L6.start
  measures "d80" radius of A6
  measures "d81" radius of A11
  measures "d82" radius of A12
  measures "d83" radius of A8
extrude "Extrude13" cut 1 faces at (-3.4167, 2.0671, 6) along direction (0, 0, -1) blind 1
extrude "Extrude14" add sketch "Sketch12" against normal blind 11 contours L2 L3 L4 A8 A9 L9 L10 L11 A11 A13 L12 L13 L15 | A2 A6 L7 L8 A10 L10 L13 L15 | A2 L1 A3 L7 L8 | A3 L2 A7 L7 L8 L9 A12 L12
extrude "Extrude15" add sketch "Sketch12" against normal blind 4 contours L0 A2 A6 L8 L10 L15 | A3 L2 L8 L9 A12 L14
sketch "Sketch13" plane through (0, -27.25, 0) normal (0, -1, 0) x (1, 0, 0)
  line L0 (2.2502, 0) -> (2.2502, 4)
  line L1 (2.2502, 4) -> (6.2013, 4)
  line L2 (6.2013, 4) -> (6.2013, 11)
  line L3 (6.2013, 11) -> (-6.2012, 11)
  line L4 (-6.2012, 11) -> (-6.2012, 0)
  line L5 (-6.2012, 0) -> (2.2502, 0)
  line L6 (-1.8, 0) -> (5.2012, 0)
  line L7 (5.2012, 11) -> (5.2012, 0)
  line L8 (6.2012, 4) -> (3.0821, 4)
  line L9 (-1.8, 11) -> (-1.8, -1.0165)
  line L10 (-1.8, 0) -> (5.2012, 0)
  line L11 (-1.8, -1.0165) -> (-1.8, 0)
  line L12 (3.85, 11) -> (5.2012, 11)
  line L13 (-0.45, 11) -> (-1.8, 11)
  arc A0 (-0.45, 11) -> (3.85, 11) centre (1.7, 11) ccw
  point P0 (1.7, 11)
  dimension "d89" = 7
  dimension "d90" = 4.3
  constraint horizontal L10
  constraint horizontal L8
  constraint coincident P0 A0.centre
  constraint coincident L6.end L7.end
  constraint perpendicular L6 L7
  constraint perpendicular L10 L11
  constraint coincident L5 L6.start
  constraint perpendicular L7 L12
  constraint perpendicular L9 L13
  measures "d89" distance of L9.end L8.end
  measures "d90" diameter of A0
sketch "Sketch14" plane through (0, 27.25, 0) normal (0, 1, 0) x (-1, 0, 0)
  line L0 (-2.2502, 4) -> (-2.2502, 0)
  line L1 (-2.2502, 0) -> (6.2013, 0)
  line L2 (6.2013, 0) -> (6.2013, 11)
  line L3 (6.2013, 11) -> (-6.2012, 11)
  line L4 (-6.2012, 11) -> (-6.2012, 4)
  line L5 (-6.2012, 4) -> (-2.2502, 4)
  line L6 (-6.2013, 0) -> (-6.2013, 4)
  line L7 (-0.8, 15) -> (-0.8, 4)
  line L8 (-6.2013, 0) -> (6.2012, 0)
  line L9 (-0.8, 15) -> (6.2012, 15)
  line L10 (6.2012, 4) -> (6.2, 4)
  line L11 (6.2012, 15) -> (6.2012, 0)
  circle A0 centre (2.7, 11) radius 2.15
  line L12 (-0.8, 4) -> (-6.2013, 4)
  line L13 (-6.2013, 0) -> (6.2012, 0)
  point P0 (2.7, 11)
  dimension "d91" = 7
  dimension "d92" = 4.3
  dimension "d137" = 12.4012
  dimension "d138" = 7
  dimension "d139" = 11
  dimension "d140" = 0.0012
  dimension "d141" = 3.5
  constraint horizontal L13
  constraint horizontal L10
  constraint collinear L10 L12
  constraint coincident P0 A0.centre
  constraint coincident L8.end L11.end
  constraint perpendicular L8 L11
  constraint coincident L6.start L8.start
  constraint perpendicular L6 L12
  constraint coincident L4.end L6.end
  constraint perpendicular L7 L12
  constraint equal L0 L6
  constraint coincident L10.start L11
  constraint perpendicular L7 L9
  constraint coincident L1 origin
  measures "d91" distance of L7.end L10.end
  measures "d92" diameter of A0
  measures "d137" distance of L4 L10.end
  measures "d138" distance of L5 P0
  measures "d139" distance of L10.start L9
  measures "d140" distance of L10.end L11
  measures "d141" distance of P0 L7
extrude "Extrude16" add sketch "Sketch13" along normal blind 8 contours L0 L1 L3 L5 L6 L7 L8 L9 L10 L12 L13 A0
extrude "Extrude17" add sketch "Sketch13" along normal blind 8 contours L0 L1 L3 L5 L6 L7 L8 L9 L10 L12 L13 A0
extrude "Extrude18" add sketch "Sketch14" along normal blind 8 contours L0 L1 L2 L3 L7 L8 L11 A0 L12 L13
extrude "Extrude19" cut 1 faces at (-2.4382, 27.25, 10.3329) along direction (0, -1, 0) blind 5
extrude "Extrude20" cut 1 faces at (1.4382, -27.25, 10.3329) along direction (0, 1, 0) blind 4
sketch "Sketch15" plane through (0, 0, 4) normal (0, 0, 1) x (-1, 0, 0)
  line L0 (-10.25, 21.2013) -> (-10.25, 10.6951)
  arc A0 (-6.2013, 12.25) -> (-10.25, 10.6951) centre (-6.2013, 6.2013) ccw
  line L1 (-6.2013, 12.25) -> (6.2013, 12.25)
  arc A1 (10.25, 10.6951) -> (6.2012, 12.25) centre (6.2013, 6.2013) ccw
  line L2 (10.25, 10.6951) -> (10.25, 21.2013)
  arc A2 (10.25, 21.2013) -> (6.2013, 25.25) centre (6.2013, 21.2013) ccw
  line L3 (6.2013, 25.25) -> (-6.2012, 25.25)
  arc A3 (-6.2012, 25.25) -> (-10.25, 21.2013) centre (-6.2012, 21.2013) ccw
  circle A4 centre (6.9428, 21.9428) radius 2
  line L4 (8.8794, 25.9428) -> (2.9428, 25.9428)
  line L5 (2.9428, 25.9428) -> (2.9428, 21.9428)
  line L6 (6.9428, 17.9428) -> (10.9428, 17.9428)
  line L7 (10.9428, 17.9428) -> (10.9428, 23.8794)
  arc A5 (2.9428, 21.9428) -> (6.9428, 17.9428) centre (6.9428, 21.9428) ccw
  line L8 (10.9428, 17.9428) -> (10.9428, 23.8794)
  line L9 (8.8794, 25.9428) -> (2.9428, 25.9428)
  line L10 (2.9428, 25.9428) -> (2.9428, 21.9428)
  line L11 (6.9428, 17.9428) -> (10.9428, 17.9428)
  arc A6 (2.9428, 21.9428) -> (6.9428, 17.9428) centre (6.9428, 21.9428) ccw
  circle A7 centre (6.9428, 21.9428) radius 2
  line L12 (-1.75, 0) -> (-22.5, 0) construction
  line L13 (0, -2.5) -> (0, -20) construction
  line L14 (-8.0247, -25.9428) -> (-2.9428, -25.9428)
  line L15 (-2.9428, -25.9428) -> (-2.9428, -21.9428)
  arc A8 (-2.9428, -21.9428) -> (-6.9428, -17.9428) centre (-6.9428, -21.9428) ccw
  line L16 (-10.9428, -17.9428) -> (-10.9428, -23.0247)
  line L17 (-6.9428, -17.9428) -> (-10.9428, -17.9428)
  circle A9 centre (-6.9428, -21.9428) radius 2
  line L18 (-8.0247, -25.9428) -> (-10.9428, -23.0247)
  line L19 (-8.0247, -25.9428) -> (-3.8978, -25.9428) construction
  line L20 (10.9428, 23.8794) -> (8.8794, 25.9428)
  point P0 (6.9428, 21.9428)
  dimension "d106" = 4
  dimension "d109" = 4
  dimension "d114" = 4
  dimension "d115" = 4
  dimension "d116" = 135
  dimension "d142" = 17.9428
  dimension "d143" = 25.9428
  dimension "d144" = 23.0247
  dimension "d145" = 5.8857
  dimension "d149" = 23.8794
  dimension "d150" = 5.9366
  dimension "d151" = 17.9428
  dimension "d152" = 8
  constraint horizontal L4
  constraint perpendicular L4 L5
  constraint parallel L4 L6
  constraint parallel L5 L7
  constraint tangent L5 A5
  constraint tangent L6 A5
  constraint horizontal L9
  constraint perpendicular L9 L10
  constraint parallel L9 L11
  constraint parallel L8 L10
  constraint tangent L10 A6
  constraint tangent L11 A6
  constraint horizontal L19
  constraint tangent A8 L17
  constraint tangent L15 A8
  constraint concentric A8 A9
  constraint concentric A5 A7
  constraint equal A5 A8
  constraint midpoint A5 A6
  constraint equal L5 L10
  constraint equal L5 L11
  constraint equal L5 L15
  constraint equal L5 L17
  constraint perpendicular L16 L17
  constraint equal L18 L19
  constraint equal A4 A9
  constraint concentric A4 A5
  constraint coincident P0 A4.centre
  measures "d106" diameter of A4
  measures "d109" radius of A5
  measures "d114" diameter of A7
  measures "d115" radius of A6
  measures "d116" angle of L18 L19
  measures "d142" distance of L12 L17
  measures "d143" distance of L12 L19
  measures "d144" distance of L12 L16.end
  measures "d145" distance of L5 L15
  measures "d149" distance of L12 L7.end
  measures "d150" distance of L5 L4.start
  measures "d151" distance of L6 L12
  measures "d152" distance of L5 L7
extrude "Extrude21" add sketch "Sketch15" along normal blind 7 contours L2 A2 L3 L5 L6 A5 L10 L11 A6 | L14 L15 A8 L16 L17 L18
chamfer "Chamfer5" distance 0.7 angle 45 2 edges at (8.8075, 21.2196, 11) (-5.0782, -22.6661, 11)
extrude "Extrude24" cut 2 faces at (3.0992, -19.4386, 4) (-3.0992, 19.4386, 4) along direction (0, 0, -1) blind 2
extrude "Extrude25" cut 1 faces at (-3.4167, 2.0671, 5) along direction (0, 0, -1) blind 3
sketch "Sketch16" plane through (0, 0, 4) normal (0, 0, 1) x (-1, 0, 0)
  arc A0 (-12.25, -21.2012) -> (-6.2012, -27.25) centre (-6.2013, -21.2012) ccw
  line L0 (-12.25, -21.2012) -> (-12.25, -43.25)
  arc A1 (-12.25, -43.25) -> (-2.2502, -43.1914) centre (-7.2501, -43.2211) ccw
  line L1 (-2.2502, -43.1914) -> (-2.2502, -35.25)
  line L2 (-2.2502, -35.25) -> (-0.8, -35.25)
  line L3 (-0.8, -35.25) -> (-0.8, -27.25)
  line L4 (-10.7579, -32.3932) -> (-6.9514, -32.3932) construction
  line L5 (-6.9514, -32.3932) -> (-6.9514, -27.9161) construction
  line L6 (-6.9514, -27.9161) -> (-10.7579, -27.9161) construction
  line L7 (-10.7579, -27.9161) -> (-10.7579, -32.3932) construction
  line L8 (-0.8, -27.25) -> (-6.2012, -27.25)
  circle A2 centre (-7.2501, -43.2211) radius 3.75
  dimension "d124" = 8
  dimension "d153" = 5.2986
  dimension "d154" = 15.3339
  dimension "d155" = 3.8065
  dimension "d156" = 4.4771
  text T0 "S" font "Arial" height 8 bold align left top in box 3.8065 x 4.4771 at (-10.7579, -32.3932) x (1, 0) y (0, 1) spacing 1 kerned
  measures "d153" distance of L0 L5
  measures "d154" distance of L0.end L6
  measures "d155" distance of L5 L7
  measures "d156" distance of L4 L6
extrude "Extrude26" add sketch "Sketch16" along normal blind 0.5 text T0
sketch "Sketch17" plane through (0, 0, 4) normal (0, 0, 1) x (-1, 0, 0)
  circle A0 centre (-7.2501, 43.2789) radius 3.75
  line L0 (-5.2012, 27.25) -> (-5.2012, 35.25)
  line L1 (-5.2012, 35.25) -> (-2.2502, 35.25)
  line L2 (-2.2502, 35.25) -> (-2.2502, 43.3086)
  arc A1 (-2.2502, 43.3086) -> (-12.25, 43.25) centre (-7.2501, 43.2789) ccw
  line L3 (-12.25, 43.25) -> (-12.25, 21.2013)
  arc A2 (-6.2013, 27.25) -> (-12.25, 21.2013) centre (-6.2012, 21.2013) ccw
  line L4 (-6.2013, 27.25) -> (-5.2012, 27.25)
  line L5 (-5.3111, 31.9604) -> (-9.1175, 31.9604) construction
  line L6 (-9.1175, 31.9604) -> (-9.1175, 27.4833) construction
  line L7 (-9.1175, 27.4833) -> (-5.3111, 27.4833) construction
  line L8 (-5.3111, 27.4833) -> (-5.3111, 31.9604) construction
  dimension "d127" = 8
  dimension "d157" = 6.9389
  dimension "d158" = 6.282
  dimension "d159" = 4.4771
  dimension "d160" = 3.8065
  text T0 "T" font "Arial" height 8 bold align left top in box 3.8065 x 4.4771 at (-5.3111, 31.9604) x (-1, 0) y (0, -1) spacing 1 kerned
  constraint vertical L8
  measures "d157" distance of L3 L8
  measures "d158" distance of L3.end L7
  measures "d159" distance of L5 L7
  measures "d160" distance of L6 L8
extrude "Extrude27" add sketch "Sketch17" along normal blind 0.5 text T0
extrude "Extrude28" cut 2 faces at (-2.0671, 10.9167, 7.5) (-2.0671, -11.5833, 7.5) along direction (0, 0, -1) blind 4
equation "d3 = ( 20.5 / 20 * 3.95 ) * 1 mm"
equation "d4 = ( 20.5 / 20 * 3.95 ) * 1 mm"
equation "d5 = ( 20.5 / 20 * 3.95 ) * 1 mm"
equation "d6 = ( 20.5 / 20 * 3.95 ) * 1 mm"
equation "d80 = ( 20.5 / 20 * 3.95 ) * 1 mm"
equation "d81 = ( 20.5 / 20 * 3.95 ) * 1 mm"
equation "d82 = ( 20.5 / 20 * 3.95 ) * 1 mm"
equation "d83 = ( 20.5 / 20 * 3.95 ) * 1 mm"

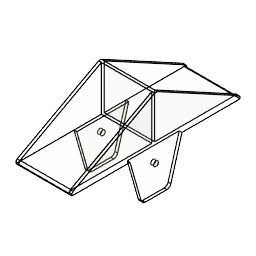
design "Bucket Receptacle (FA1)"
Autodesk Fusion 360 part; units mm, degrees
sketch "Sketch1" plane through (0, 0, 0) normal (0, 0, 1) x (1, 0, 0)
  line L0 (20, 60) -> (-20, 60)
  line L1 (-20, 60) -> (-20, -60)
  line L2 (-20, -60) -> (20, -60)
  line L3 (20, -60) -> (20, 60)
  line L4 (20, 60) -> (-20, -60) construction
  line L5 (-20, 60) -> (20, -60) construction
  dimension "d1" = 40
  dimension "d2" = 120
  constraint horizontal L0
  constraint perpendicular L0 L1
  constraint parallel L0 L2
  constraint parallel L1 L3
  constraint coincident L4 origin
  constraint coincident L5 origin
  measures "d1" distance of L1.end L2.end
  measures "d2" distance of L0.end L1.end
extrude "Extrude1" add sketch "Sketch1" along normal blind 2
sketch "Sketch2" plane through (0, 0, 0) normal (1, 0, 0) x (0, 1, 0)
  line L0 (-1, 2) -> (1, 2)
  line L1 (1, 2) -> (1, 34)
  line L2 (1, 34) -> (-1, 34)
  line L3 (-1, 34) -> (-1, 2)
  line L4 (-60, 2) -> (-1, 34)
  line L5 (-60, 2) -> (-1, 2)
  line L6 (1, 34) -> (60, 2)
  line L7 (1, 2) -> (60, 2)
  dimension "d5" = 32
  dimension "d16" = 2
  dimension "d25" = 1
  dimension "d26" = 60
  dimension "d27" = 2
  constraint horizontal L0
  constraint vertical L1
  constraint horizontal L2
  constraint vertical L3
  constraint perpendicular L3 L5
  constraint perpendicular L1 L7
  constraint equal L5 L7
  measures "d5" distance of L0.start L2.end
  measures "d16" distance of L0.start L0.end
  measures "d25" distance of origin L3
  measures "d26" horizontal distance of origin L6.end
  measures "d27" distance of origin L0
sketch "Sketch3" plane through (0, 0, 0) normal (1, 0, 0) x (0, 1, 0)
  line L0 (0, 0) -> (0, -30) construction
  line L1 (0, 0) -> (0, -10) construction
  circle A0 centre (0, -10) radius 1.75
  line L2 (0, -30) -> (-7.7353, -30)
  line L3 (-10.6205, -27.8219) -> (-18.5463, 0)
  line L4 (0, -30) -> (7.7353, -30)
  line L5 (10.6205, -27.8219) -> (18.5463, 0)
  line L6 (18.5463, 0) -> (-18.5463, 0)
  arc A1 (7.7353, -30) -> (10.6205, -27.8219) centre (7.7353, -27) ccw
  arc A2 (-10.6205, -27.8219) -> (-7.7353, -30) centre (-7.7353, -27) ccw
  dimension "d21" = 10
  dimension "d22" = 3.5
  dimension "d23" = 30
  dimension "d24" = 3
  dimension "d28" = 18.5463
  dimension "d29" = 74.099
  constraint coincident L0.start L1.start
  constraint vertical L0
  constraint coincident L1.end A0.centre
  constraint perpendicular L0 L2
  constraint symmetric L2.start L0 L4.start
  constraint symmetric L0 L3.end L5.end
  constraint tangent L4 A1
  constraint tangent L5 A1
  constraint tangent L2 A2
  constraint tangent L3 A2
  constraint equal A1 A2
  constraint vertical L0.start L1.end
  constraint symmetric L0 L5.start L3.start
  constraint coincident L0.start L6
  measures "d21" distance of L0.start L1.end
  measures "d22" diameter of A0
  measures "d23" distance of L0.start L0.end
  measures "d24" radius of A1
  measures "d28" distance of L0 L3.end
  measures "d29" angle of L5 L6
extrude "Extrude2" add sketch "Sketch2" along normal up to surface (20 mm away) and the other way up to surface (20 mm away) contours L0 L1 L2 L3
extrude "Extrude3" add sketch "Sketch2" sketch "Sketch3" against normal blind 2 of sketch 2 start surface through (20, -60, 0) normal (1, 0, 0)
extrude "Extrude4" add sketch "Sketch2" sketch "Sketch3" along normal blind 2 of sketch 2 start surface through (-20, 60, 0) normal (-1, 0, 0)
fillet "Fillet1" radius 1.5 6 edges at (0, 60, 2) (19, 60, 2) (-19, 60, 2) (0, -60, 2) (19, -60, 2) (-19, -60, 2)

design "LB1 - Baseplate"
Autodesk Fusion 360 part; units mm, degrees